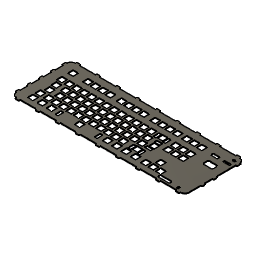
Plate v20 (Autodesk Fusion 360 design; units mm, degrees)
Autodesk Fusion 360 part; units mm, degrees
note: some values were not read from the file. Set by a fixed rule: which sketch regions a step uses.
(part 1 of 3)
sketch "Sketch1" plane through (0, 0, 0) normal (0, 0, 1) x (1, 0, 0)
  line L0 (3.025, -2.525) -> (16.025, -2.525)
  line L1 (3.025, -16.525) -> (16.025, -16.525)
  line L2 (2.525, -3.025) -> (2.525, -16.025)
  line L3 (16.525, -3.025) -> (16.525, -16.025)
  arc A0 (3.025, -2.525) -> (2.525, -3.025) centre (3.025, -3.025) ccw
  arc A1 (16.525, -3.025) -> (16.025, -2.525) centre (16.025, -3.025) ccw
  arc A2 (2.525, -16.025) -> (3.025, -16.525) centre (3.025, -16.025) ccw
  arc A3 (16.025, -16.525) -> (16.525, -16.025) centre (16.025, -16.025) ccw
  line L4 (41.125, -2.525) -> (54.125, -2.525)
  line L5 (41.125, -16.525) -> (54.125, -16.525)
  line L6 (40.625, -3.025) -> (40.625, -16.025)
  line L7 (54.625, -3.025) -> (54.625, -16.025)
  arc A4 (41.125, -2.525) -> (40.625, -3.025) centre (41.125, -3.025) ccw
  arc A5 (54.625, -3.025) -> (54.125, -2.525) centre (54.125, -3.025) ccw
  arc A6 (40.625, -16.025) -> (41.125, -16.525) centre (41.125, -16.025) ccw
  arc A7 (54.125, -16.525) -> (54.625, -16.025) centre (54.125, -16.025) ccw
  line L8 (60.175, -2.525) -> (73.175, -2.525)
  line L9 (60.175, -16.525) -> (73.175, -16.525)
  line L10 (59.675, -3.025) -> (59.675, -16.025)
  line L11 (73.675, -3.025) -> (73.675, -16.025)
  arc A8 (60.175, -2.525) -> (59.675, -3.025) centre (60.175, -3.025) ccw
  arc A9 (73.675, -3.025) -> (73.175, -2.525) centre (73.175, -3.025) ccw
  arc A10 (59.675, -16.025) -> (60.175, -16.525) centre (60.175, -16.025) ccw
  arc A11 (73.175, -16.525) -> (73.675, -16.025) centre (73.175, -16.025) ccw
  line L12 (79.225, -2.525) -> (92.225, -2.525)
  line L13 (79.225, -16.525) -> (92.225, -16.525)
  line L14 (78.725, -3.025) -> (78.725, -16.025)
  line L15 (92.725, -3.025) -> (92.725, -16.025)
  arc A12 (79.225, -2.525) -> (78.725, -3.025) centre (79.225, -3.025) ccw
  arc A13 (92.725, -3.025) -> (92.225, -2.525) centre (92.225, -3.025) ccw
  arc A14 (78.725, -16.025) -> (79.225, -16.525) centre (79.225, -16.025) ccw
  arc A15 (92.225, -16.525) -> (92.725, -16.025) centre (92.225, -16.025) ccw
  line L16 (98.275, -2.525) -> (111.275, -2.525)
  line L17 (98.275, -16.525) -> (111.275, -16.525)
  line L18 (97.775, -3.025) -> (97.775, -16.025)
  line L19 (111.775, -3.025) -> (111.775, -16.025)
  arc A16 (98.275, -2.525) -> (97.775, -3.025) centre (98.275, -3.025) ccw
  arc A17 (111.775, -3.025) -> (111.275, -2.525) centre (111.275, -3.025) ccw
  arc A18 (97.775, -16.025) -> (98.275, -16.525) centre (98.275, -16.025) ccw
  arc A19 (111.275, -16.525) -> (111.775, -16.025) centre (111.275, -16.025) ccw
  line L20 (126.85, -2.525) -> (139.85, -2.525)
  line L21 (126.85, -16.525) -> (139.85, -16.525)
  line L22 (126.35, -3.025) -> (126.35, -16.025)
  line L23 (140.35, -3.025) -> (140.35, -16.025)
  arc A20 (126.85, -2.525) -> (126.35, -3.025) centre (126.85, -3.025) ccw
  arc A21 (140.35, -3.025) -> (139.85, -2.525) centre (139.85, -3.025) ccw
  arc A22 (126.35, -16.025) -> (126.85, -16.525) centre (126.85, -16.025) ccw
  arc A23 (139.85, -16.525) -> (140.35, -16.025) centre (139.85, -16.025) ccw
  line L24 (145.9, -2.525) -> (158.9, -2.525)
  line L25 (145.9, -16.525) -> (158.9, -16.525)
  line L26 (145.4, -3.025) -> (145.4, -16.025)
  line L27 (159.4, -3.025) -> (159.4, -16.025)
  arc A24 (145.9, -2.525) -> (145.4, -3.025) centre (145.9, -3.025) ccw
  arc A25 (159.4, -3.025) -> (158.9, -2.525) centre (158.9, -3.025) ccw
  arc A26 (145.4, -16.025) -> (145.9, -16.525) centre (145.9, -16.025) ccw
  arc A27 (158.9, -16.525) -> (159.4, -16.025) centre (158.9, -16.025) ccw
  line L28 (164.95, -2.525) -> (177.95, -2.525)
  line L29 (164.95, -16.525) -> (177.95, -16.525)
  line L30 (164.45, -3.025) -> (164.45, -16.025)
  line L31 (178.45, -3.025) -> (178.45, -16.025)
  arc A28 (164.95, -2.525) -> (164.45, -3.025) centre (164.95, -3.025) ccw
  arc A29 (178.45, -3.025) -> (177.95, -2.525) centre (177.95, -3.025) ccw
  arc A30 (164.45, -16.025) -> (164.95, -16.525) centre (164.95, -16.025) ccw
  arc A31 (177.95, -16.525) -> (178.45, -16.025) centre (177.95, -16.025) ccw
  line L32 (184, -2.525) -> (197, -2.525)
  line L33 (184, -16.525) -> (197, -16.525)
  line L34 (183.5, -3.025) -> (183.5, -16.025)
  line L35 (197.5, -3.025) -> (197.5, -16.025)
  arc A32 (184, -2.525) -> (183.5, -3.025) centre (184, -3.025) ccw
  arc A33 (197.5, -3.025) -> (197, -2.525) centre (197, -3.025) ccw
  arc A34 (183.5, -16.025) -> (184, -16.525) centre (184, -16.025) ccw
  arc A35 (197, -16.525) -> (197.5, -16.025) centre (197, -16.025) ccw
  line L36 (212.575, -2.525) -> (225.575, -2.525)
  line L37 (212.575, -16.525) -> (225.575, -16.525)
  line L38 (212.075, -3.025) -> (212.075, -16.025)
  line L39 (226.075, -3.025) -> (226.075, -16.025)
  arc A36 (212.575, -2.525) -> (212.075, -3.025) centre (212.575, -3.025) ccw
  arc A37 (226.075, -3.025) -> (225.575, -2.525) centre (225.575, -3.025) ccw
  arc A38 (212.075, -16.025) -> (212.575, -16.525) centre (212.575, -16.025) ccw
  arc A39 (225.575, -16.525) -> (226.075, -16.025) centre (225.575, -16.025) ccw
  line L40 (231.625, -2.525) -> (244.625, -2.525)
  line L41 (231.625, -16.525) -> (244.625, -16.525)
  line L42 (231.125, -3.025) -> (231.125, -16.025)
  line L43 (245.125, -3.025) -> (245.125, -16.025)
  arc A40 (231.625, -2.525) -> (231.125, -3.025) centre (231.625, -3.025) ccw
  arc A41 (245.125, -3.025) -> (244.625, -2.525) centre (244.625, -3.025) ccw
  arc A42 (231.125, -16.025) -> (231.625, -16.525) centre (231.625, -16.025) ccw
  arc A43 (244.625, -16.525) -> (245.125, -16.025) centre (244.625, -16.025) ccw
  line L44 (250.675, -2.525) -> (263.675, -2.525)
  line L45 (250.675, -16.525) -> (263.675, -16.525)
  line L46 (250.175, -3.025) -> (250.175, -16.025)
  line L47 (264.175, -3.025) -> (264.175, -16.025)
  arc A44 (250.675, -2.525) -> (250.175, -3.025) centre (250.675, -3.025) ccw
  arc A45 (264.175, -3.025) -> (263.675, -2.525) centre (263.675, -3.025) ccw
  arc A46 (250.175, -16.025) -> (250.675, -16.525) centre (250.675, -16.025) ccw
  arc A47 (263.675, -16.525) -> (264.175, -16.025) centre (263.675, -16.025) ccw
  line L48 (269.725, -2.525) -> (282.725, -2.525)
  line L49 (269.725, -16.525) -> (282.725, -16.525)
  line L50 (269.225, -3.025) -> (269.225, -16.025)
  line L51 (283.225, -3.025) -> (283.225, -16.025)
  arc A48 (269.725, -2.525) -> (269.225, -3.025) centre (269.725, -3.025) ccw
  arc A49 (283.225, -3.025) -> (282.725, -2.525) centre (282.725, -3.025) ccw
  arc A50 (269.225, -16.025) -> (269.725, -16.525) centre (269.725, -16.025) ccw
  arc A51 (282.725, -16.525) -> (283.225, -16.025) centre (282.725, -16.025) ccw
  line L52 (293.5375, -2.525) -> (306.5375, -2.525)
  line L53 (293.5375, -16.525) -> (306.5375, -16.525)
  line L54 (293.0375, -3.025) -> (293.0375, -16.025)
  line L55 (307.0375, -3.025) -> (307.0375, -16.025)
  arc A52 (293.5375, -2.525) -> (293.0375, -3.025) centre (293.5375, -3.025) ccw
  arc A53 (307.0375, -3.025) -> (306.5375, -2.525) centre (306.5375, -3.025) ccw
  arc A54 (293.0375, -16.025) -> (293.5375, -16.525) centre (293.5375, -16.025) ccw
  arc A55 (306.5375, -16.525) -> (307.0375, -16.025) centre (306.5375, -16.025) ccw
  line L56 (312.5875, -2.525) -> (325.5875, -2.525)
  line L57 (312.5875, -16.525) -> (325.5875, -16.525)
  line L58 (312.0875, -3.025) -> (312.0875, -16.025)
  line L59 (326.0875, -3.025) -> (326.0875, -16.025)
  arc A56 (312.5875, -2.525) -> (312.0875, -3.025) centre (312.5875, -3.025) ccw
  arc A57 (326.0875, -3.025) -> (325.5875, -2.525) centre (325.5875, -3.025) ccw
  arc A58 (312.0875, -16.025) -> (312.5875, -16.525) centre (312.5875, -16.025) ccw
  arc A59 (325.5875, -16.525) -> (326.0875, -16.025) centre (325.5875, -16.025) ccw
  line L60 (331.6375, -2.525) -> (344.6375, -2.525)
  line L61 (331.6375, -16.525) -> (344.6375, -16.525)
  line L62 (331.1375, -3.025) -> (331.1375, -16.025)
  line L63 (345.1375, -3.025) -> (345.1375, -16.025)
  arc A60 (331.6375, -2.525) -> (331.1375, -3.025) centre (331.6375, -3.025) ccw
  arc A61 (345.1375, -3.025) -> (344.6375, -2.525) centre (344.6375, -3.025) ccw
  arc A62 (331.1375, -16.025) -> (331.6375, -16.525) centre (331.6375, -16.025) ccw
  arc A63 (344.6375, -16.525) -> (345.1375, -16.025) centre (344.6375, -16.025) ccw
  line L64 (3.025, -31.1) -> (16.025, -31.1)
  line L65 (3.025, -45.1) -> (16.025, -45.1)
  line L66 (2.525, -31.6) -> (2.525, -44.6)
  line L67 (16.525, -31.6) -> (16.525, -44.6)
  arc A64 (3.025, -31.1) -> (2.525, -31.6) centre (3.025, -31.6) ccw
  arc A65 (16.525, -31.6) -> (16.025, -31.1) centre (16.025, -31.6) ccw
  arc A66 (2.525, -44.6) -> (3.025, -45.1) centre (3.025, -44.6) ccw
  arc A67 (16.025, -45.1) -> (16.525, -44.6) centre (16.025, -44.6) ccw
  line L68 (22.075, -31.1) -> (35.075, -31.1)
  line L69 (22.075, -45.1) -> (35.075, -45.1)
  line L70 (21.575, -31.6) -> (21.575, -44.6)
  line L71 (35.575, -31.6) -> (35.575, -44.6)
  arc A68 (22.075, -31.1) -> (21.575, -31.6) centre (22.075, -31.6) ccw
  arc A69 (35.575, -31.6) -> (35.075, -31.1) centre (35.075, -31.6) ccw
  arc A70 (21.575, -44.6) -> (22.075, -45.1) centre (22.075, -44.6) ccw
  arc A71 (35.075, -45.1) -> (35.575, -44.6) centre (35.075, -44.6) ccw
  line L72 (41.125, -31.1) -> (54.125, -31.1)
  line L73 (41.125, -45.1) -> (54.125, -45.1)
  line L74 (40.625, -31.6) -> (40.625, -44.6)
  line L75 (54.625, -31.6) -> (54.625, -44.6)
  arc A72 (41.125, -31.1) -> (40.625, -31.6) centre (41.125, -31.6) ccw
  arc A73 (54.625, -31.6) -> (54.125, -31.1) centre (54.125, -31.6) ccw
  arc A74 (40.625, -44.6) -> (41.125, -45.1) centre (41.125, -44.6) ccw
  arc A75 (54.125, -45.1) -> (54.625, -44.6) centre (54.125, -44.6) ccw
  line L76 (60.175, -31.1) -> (73.175, -31.1)
  line L77 (60.175, -45.1) -> (73.175, -45.1)
  line L78 (59.675, -31.6) -> (59.675, -44.6)
  line L79 (73.675, -31.6) -> (73.675, -44.6)
  arc A76 (60.175, -31.1) -> (59.675, -31.6) centre (60.175, -31.6) ccw
  arc A77 (73.675, -31.6) -> (73.175, -31.1) centre (73.175, -31.6) ccw
  arc A78 (59.675, -44.6) -> (60.175, -45.1) centre (60.175, -44.6) ccw
  arc A79 (73.175, -45.1) -> (73.675, -44.6) centre (73.175, -44.6) ccw
  line L80 (79.225, -31.1) -> (92.225, -31.1)
  line L81 (79.225, -45.1) -> (92.225, -45.1)
  line L82 (78.725, -31.6) -> (78.725, -44.6)
  line L83 (92.725, -31.6) -> (92.725, -44.6)
  arc A80 (79.225, -31.1) -> (78.725, -31.6) centre (79.225, -31.6) ccw
  arc A81 (92.725, -31.6) -> (92.225, -31.1) centre (92.225, -31.6) ccw
  arc A82 (78.725, -44.6) -> (79.225, -45.1) centre (79.225, -44.6) ccw
  arc A83 (92.225, -45.1) -> (92.725, -44.6) centre (92.225, -44.6) ccw
  line L84 (98.275, -31.1) -> (111.275, -31.1)
  line L85 (98.275, -45.1) -> (111.275, -45.1)
  line L86 (97.775, -31.6) -> (97.775, -44.6)
  line L87 (111.775, -31.6) -> (111.775, -44.6)
  arc A84 (98.275, -31.1) -> (97.775, -31.6) centre (98.275, -31.6) ccw
  arc A85 (111.775, -31.6) -> (111.275, -31.1) centre (111.275, -31.6) ccw
  arc A86 (97.775, -44.6) -> (98.275, -45.1) centre (98.275, -44.6) ccw
  arc A87 (111.275, -45.1) -> (111.775, -44.6) centre (111.275, -44.6) ccw
  line L88 (117.325, -31.1) -> (130.325, -31.1)
  line L89 (117.325, -45.1) -> (130.325, -45.1)
  line L90 (116.825, -31.6) -> (116.825, -44.6)
  line L91 (130.825, -31.6) -> (130.825, -44.6)
  arc A88 (117.325, -31.1) -> (116.825, -31.6) centre (117.325, -31.6) ccw
  arc A89 (130.825, -31.6) -> (130.325, -31.1) centre (130.325, -31.6) ccw
  arc A90 (116.825, -44.6) -> (117.325, -45.1) centre (117.325, -44.6) ccw
  arc A91 (130.325, -45.1) -> (130.825, -44.6) centre (130.325, -44.6) ccw
  line L92 (136.375, -31.1) -> (149.375, -31.1)
  line L93 (136.375, -45.1) -> (149.375, -45.1)
  line L94 (135.875, -31.6) -> (135.875, -44.6)
  line L95 (149.875, -31.6) -> (149.875, -44.6)
  arc A92 (136.375, -31.1) -> (135.875, -31.6) centre (136.375, -31.6) ccw
  arc A93 (149.875, -31.6) -> (149.375, -31.1) centre (149.375, -31.6) ccw
  arc A94 (135.875, -44.6) -> (136.375, -45.1) centre (136.375, -44.6) ccw
  arc A95 (149.375, -45.1) -> (149.875, -44.6) centre (149.375, -44.6) ccw
  line L96 (155.425, -31.1) -> (168.425, -31.1)
  line L97 (155.425, -45.1) -> (168.425, -45.1)
  line L98 (154.925, -31.6) -> (154.925, -44.6)
  line L99 (168.925, -31.6) -> (168.925, -44.6)
  arc A96 (155.425, -31.1) -> (154.925, -31.6) centre (155.425, -31.6) ccw
  arc A97 (168.925, -31.6) -> (168.425, -31.1) centre (168.425, -31.6) ccw
  arc A98 (154.925, -44.6) -> (155.425, -45.1) centre (155.425, -44.6) ccw
  arc A99 (168.425, -45.1) -> (168.925, -44.6) centre (168.425, -44.6) ccw
  line L100 (174.475, -31.1) -> (187.475, -31.1)
  line L101 (174.475, -45.1) -> (187.475, -45.1)
  line L102 (173.975, -31.6) -> (173.975, -44.6)
  line L103 (187.975, -31.6) -> (187.975, -44.6)
  arc A100 (174.475, -31.1) -> (173.975, -31.6) centre (174.475, -31.6) ccw
  arc A101 (187.975, -31.6) -> (187.475, -31.1) centre (187.475, -31.6) ccw
  arc A102 (173.975, -44.6) -> (174.475, -45.1) centre (174.475, -44.6) ccw
  arc A103 (187.475, -45.1) -> (187.975, -44.6) centre (187.475, -44.6) ccw
  line L104 (193.525, -31.1) -> (206.525, -31.1)
  line L105 (193.525, -45.1) -> (206.525, -45.1)
  line L106 (193.025, -31.6) -> (193.025, -44.6)
  line L107 (207.025, -31.6) -> (207.025, -44.6)
  arc A104 (193.525, -31.1) -> (193.025, -31.6) centre (193.525, -31.6) ccw
  arc A105 (207.025, -31.6) -> (206.525, -31.1) centre (206.525, -31.6) ccw
  arc A106 (193.025, -44.6) -> (193.525, -45.1) centre (193.525, -44.6) ccw
  arc A107 (206.525, -45.1) -> (207.025, -44.6) centre (206.525, -44.6) ccw
  line L108 (212.575, -31.1) -> (225.575, -31.1)
  line L109 (212.575, -45.1) -> (225.575, -45.1)
  line L110 (212.075, -31.6) -> (212.075, -44.6)
  line L111 (226.075, -31.6) -> (226.075, -44.6)
  arc A108 (212.575, -31.1) -> (212.075, -31.6) centre (212.575, -31.6) ccw
  arc A109 (226.075, -31.6) -> (225.575, -31.1) centre (225.575, -31.6) ccw
  arc A110 (212.075, -44.6) -> (212.575, -45.1) centre (212.575, -44.6) ccw
  arc A111 (225.575, -45.1) -> (226.075, -44.6) centre (225.575, -44.6) ccw
  line L112 (231.625, -31.1) -> (244.625, -31.1)
  line L113 (231.625, -45.1) -> (244.625, -45.1)
  line L114 (231.125, -31.6) -> (231.125, -44.6)
  line L115 (245.125, -31.6) -> (245.125, -44.6)
  arc A112 (231.625, -31.1) -> (231.125, -31.6) centre (231.625, -31.6) ccw
  arc A113 (245.125, -31.6) -> (244.625, -31.1) centre (244.625, -31.6) ccw
  arc A114 (231.125, -44.6) -> (231.625, -45.1) centre (231.625, -44.6) ccw
  arc A115 (244.625, -45.1) -> (245.125, -44.6) centre (244.625, -44.6) ccw
  line L116 (260.2, -31.1) -> (273.2, -31.1)
  line L117 (260.2, -45.1) -> (273.2, -45.1)
  line L118 (259.7, -31.6) -> (259.7, -44.6)
  line L119 (273.7, -31.6) -> (273.7, -44.6)
  arc A116 (260.2, -31.1) -> (259.7, -31.6) centre (260.2, -31.6) ccw
  arc A117 (273.7, -31.6) -> (273.2, -31.1) centre (273.2, -31.6) ccw
  arc A118 (259.7, -44.6) -> (260.2, -45.1) centre (260.2, -44.6) ccw
  arc A119 (273.2, -45.1) -> (273.7, -44.6) centre (273.2, -44.6) ccw
  line L120 (251.762, -32.1) -> (257.762, -32.1)
  line L121 (251.762, -47.1) -> (257.762, -47.1)
  line L122 (251.262, -32.6) -> (251.262, -46.6)
  line L123 (258.262, -32.6) -> (258.262, -46.6)
  arc A120 (251.762, -32.1) -> (251.262, -32.6) centre (251.762, -32.6) ccw
  arc A121 (258.262, -32.6) -> (257.762, -32.1) centre (257.762, -32.6) ccw
  arc A122 (251.262, -46.6) -> (251.762, -47.1) centre (251.762, -46.6) ccw
  arc A123 (257.762, -47.1) -> (258.262, -46.6) centre (257.762, -46.6) ccw
  line L124 (275.638, -32.1) -> (281.638, -32.1)
  line L125 (275.638, -47.1) -> (281.638, -47.1)
  line L126 (275.138, -32.6) -> (275.138, -46.6)
  line L127 (282.138, -32.6) -> (282.138, -46.6)
  arc A124 (275.638, -32.1) -> (275.138, -32.6) centre (275.638, -32.6) ccw
  arc A125 (282.138, -32.6) -> (281.638, -32.1) centre (281.638, -32.6) ccw
  arc A126 (275.138, -46.6) -> (275.638, -47.1) centre (275.638, -46.6) ccw
  arc A127 (281.638, -47.1) -> (282.138, -46.6) centre (281.638, -46.6) ccw
  line L128 (293.5375, -31.1) -> (306.5375, -31.1)
  line L129 (293.5375, -45.1) -> (306.5375, -45.1)
  line L130 (293.0375, -31.6) -> (293.0375, -44.6)
  line L131 (307.0375, -31.6) -> (307.0375, -44.6)
  arc A128 (293.5375, -31.1) -> (293.0375, -31.6) centre (293.5375, -31.6) ccw
  arc A129 (307.0375, -31.6) -> (306.5375, -31.1) centre (306.5375, -31.6) ccw
  arc A130 (293.0375, -44.6) -> (293.5375, -45.1) centre (293.5375, -44.6) ccw
  arc A131 (306.5375, -45.1) -> (307.0375, -44.6) centre (306.5375, -44.6) ccw
  line L132 (312.5875, -31.1) -> (325.5875, -31.1)
  line L133 (312.5875, -45.1) -> (325.5875, -45.1)
  line L134 (312.0875, -31.6) -> (312.0875, -44.6)
  line L135 (326.0875, -31.6) -> (326.0875, -44.6)
  arc A132 (312.5875, -31.1) -> (312.0875, -31.6) centre (312.5875, -31.6) ccw
  arc A133 (326.0875, -31.6) -> (325.5875, -31.1) centre (325.5875, -31.6) ccw
  arc A134 (312.0875, -44.6) -> (312.5875, -45.1) centre (312.5875, -44.6) ccw
  arc A135 (325.5875, -45.1) -> (326.0875, -44.6) centre (325.5875, -44.6) ccw
  line L136 (331.6375, -31.1) -> (344.6375, -31.1)
  line L137 (331.6375, -45.1) -> (344.6375, -45.1)
  line L138 (331.1375, -31.6) -> (331.1375, -44.6)
  line L139 (345.1375, -31.6) -> (345.1375, -44.6)
  arc A136 (331.6375, -31.1) -> (331.1375, -31.6) centre (331.6375, -31.6) ccw
  arc A137 (345.1375, -31.6) -> (344.6375, -31.1) centre (344.6375, -31.6) ccw
  arc A138 (331.1375, -44.6) -> (331.6375, -45.1) centre (331.6375, -44.6) ccw
  arc A139 (344.6375, -45.1) -> (345.1375, -44.6) centre (344.6375, -44.6) ccw
  line L140 (7.7875, -50.15) -> (20.7875, -50.15)
  line L141 (7.7875, -64.15) -> (20.7875, -64.15)
  line L142 (7.2875, -50.65) -> (7.2875, -63.65)
  line L143 (21.2875, -50.65) -> (21.2875, -63.65)
  arc A140 (7.7875, -50.15) -> (7.2875, -50.65) centre (7.7875, -50.65) ccw
  arc A141 (21.2875, -50.65) -> (20.7875, -50.15) centre (20.7875, -50.65) ccw
  arc A142 (7.2875, -63.65) -> (7.7875, -64.15) centre (7.7875, -63.65) ccw
  arc A143 (20.7875, -64.15) -> (21.2875, -63.65) centre (20.7875, -63.65) ccw
  line L144 (31.6, -50.15) -> (44.6, -50.15)
  line L145 (31.6, -64.15) -> (44.6, -64.15)
  line L146 (31.1, -50.65) -> (31.1, -63.65)
  line L147 (45.1, -50.65) -> (45.1, -63.65)
  arc A144 (31.6, -50.15) -> (31.1, -50.65) centre (31.6, -50.65) ccw
  arc A145 (45.1, -50.65) -> (44.6, -50.15) centre (44.6, -50.65) ccw
  arc A146 (31.1, -63.65) -> (31.6, -64.15) centre (31.6, -63.65) ccw
  arc A147 (44.6, -64.15) -> (45.1, -63.65) centre (44.6, -63.65) ccw
  line L148 (50.65, -50.15) -> (63.65, -50.15)
  line L149 (50.65, -64.15) -> (63.65, -64.15)
  line L150 (50.15, -50.65) -> (50.15, -63.65)
  line L151 (64.15, -50.65) -> (64.15, -63.65)
  arc A148 (50.65, -50.15) -> (50.15, -50.65) centre (50.65, -50.65) ccw
  arc A149 (64.15, -50.65) -> (63.65, -50.15) centre (63.65, -50.65) ccw
  arc A150 (50.15, -63.65) -> (50.65, -64.15) centre (50.65, -63.65) ccw
  arc A151 (63.65, -64.15) -> (64.15, -63.65) centre (63.65, -63.65) ccw
  line L152 (69.7, -50.15) -> (82.7, -50.15)
  line L153 (69.7, -64.15) -> (82.7, -64.15)
  line L154 (69.2, -50.65) -> (69.2, -63.65)
  line L155 (83.2, -50.65) -> (83.2, -63.65)
  arc A152 (69.7, -50.15) -> (69.2, -50.65) centre (69.7, -50.65) ccw
  arc A153 (83.2, -50.65) -> (82.7, -50.15) centre (82.7, -50.65) ccw
  arc A154 (69.2, -63.65) -> (69.7, -64.15) centre (69.7, -63.65) ccw
  arc A155 (82.7, -64.15) -> (83.2, -63.65) centre (82.7, -63.65) ccw
  line L156 (88.75, -50.15) -> (101.75, -50.15)
  line L157 (88.75, -64.15) -> (101.75, -64.15)
  line L158 (88.25, -50.65) -> (88.25, -63.65)
  line L159 (102.25, -50.65) -> (102.25, -63.65)
  arc A156 (88.75, -50.15) -> (88.25, -50.65) centre (88.75, -50.65) ccw
  arc A157 (102.25, -50.65) -> (101.75, -50.15) centre (101.75, -50.65) ccw
  arc A158 (88.25, -63.65) -> (88.75, -64.15) centre (88.75, -63.65) ccw
  arc A159 (101.75, -64.15) -> (102.25, -63.65) centre (101.75, -63.65) ccw
  line L160 (107.8, -50.15) -> (120.8, -50.15)
  line L161 (107.8, -64.15) -> (120.8, -64.15)
  line L162 (107.3, -50.65) -> (107.3, -63.65)
  line L163 (121.3, -50.65) -> (121.3, -63.65)
  arc A160 (107.8, -50.15) -> (107.3, -50.65) centre (107.8, -50.65) ccw
  arc A161 (121.3, -50.65) -> (120.8, -50.15) centre (120.8, -50.65) ccw
  arc A162 (107.3, -63.65) -> (107.8, -64.15) centre (107.8, -63.65) ccw
  arc A163 (120.8, -64.15) -> (121.3, -63.65) centre (120.8, -63.65) ccw
  line L164 (126.85, -50.15) -> (139.85, -50.15)
  line L165 (126.85, -64.15) -> (139.85, -64.15)
  line L166 (126.35, -50.65) -> (126.35, -63.65)
  line L167 (140.35, -50.65) -> (140.35, -63.65)
  arc A164 (126.85, -50.15) -> (126.35, -50.65) centre (126.85, -50.65) ccw
  arc A165 (140.35, -50.65) -> (139.85, -50.15) centre (139.85, -50.65) ccw
  arc A166 (126.35, -63.65) -> (126.85, -64.15) centre (126.85, -63.65) ccw
  arc A167 (139.85, -64.15) -> (140.35, -63.65) centre (139.85, -63.65) ccw
  line L168 (145.9, -50.15) -> (158.9, -50.15)
  line L169 (145.9, -64.15) -> (158.9, -64.15)
  line L170 (145.4, -50.65) -> (145.4, -63.65)
  line L171 (159.4, -50.65) -> (159.4, -63.65)
  arc A168 (145.9, -50.15) -> (145.4, -50.65) centre (145.9, -50.65) ccw
  arc A169 (159.4, -50.65) -> (158.9, -50.15) centre (158.9, -50.65) ccw
  arc A170 (145.4, -63.65) -> (145.9, -64.15) centre (145.9, -63.65) ccw
  arc A171 (158.9, -64.15) -> (159.4, -63.65) centre (158.9, -63.65) ccw
  line L172 (164.95, -50.15) -> (177.95, -50.15)
  line L173 (164.95, -64.15) -> (177.95, -64.15)
  line L174 (164.45, -50.65) -> (164.45, -63.65)
  line L175 (178.45, -50.65) -> (178.45, -63.65)
  arc A172 (164.95, -50.15) -> (164.45, -50.65) centre (164.95, -50.65) ccw
  arc A173 (178.45, -50.65) -> (177.95, -50.15) centre (177.95, -50.65) ccw
  arc A174 (164.45, -63.65) -> (164.95, -64.15) centre (164.95, -63.65) ccw
  arc A175 (177.95, -64.15) -> (178.45, -63.65) centre (177.95, -63.65) ccw
  line L176 (184, -50.15) -> (197, -50.15)
  line L177 (184, -64.15) -> (197, -64.15)
  line L178 (183.5, -50.65) -> (183.5, -63.65)
  line L179 (197.5, -50.65) -> (197.5, -63.65)
  arc A176 (184, -50.15) -> (183.5, -50.65) centre (184, -50.65) ccw
  arc A177 (197.5, -50.65) -> (197, -50.15) centre (197, -50.65) ccw
  arc A178 (183.5, -63.65) -> (184, -64.15) centre (184, -63.65) ccw
  arc A179 (197, -64.15) -> (197.5, -63.65) centre (197, -63.65) ccw
  line L180 (203.05, -50.15) -> (216.05, -50.15)
  line L181 (203.05, -64.15) -> (216.05, -64.15)
  line L182 (202.55, -50.65) -> (202.55, -63.65)
  line L183 (216.55, -50.65) -> (216.55, -63.65)
  arc A180 (203.05, -50.15) -> (202.55, -50.65) centre (203.05, -50.65) ccw
  arc A181 (216.55, -50.65) -> (216.05, -50.15) centre (216.05, -50.65) ccw
  arc A182 (202.55, -63.65) -> (203.05, -64.15) centre (203.05, -63.65) ccw
  arc A183 (216.05, -64.15) -> (216.55, -63.65) centre (216.05, -63.65) ccw
  line L184 (222.1, -50.15) -> (235.1, -50.15)
  line L185 (222.1, -64.15) -> (235.1, -64.15)
  line L186 (221.6, -50.65) -> (221.6, -63.65)
  line L187 (235.6, -50.65) -> (235.6, -63.65)
  arc A184 (222.1, -50.15) -> (221.6, -50.65) centre (222.1, -50.65) ccw
  arc A185 (235.6, -50.65) -> (235.1, -50.15) centre (235.1, -50.65) ccw
  arc A186 (221.6, -63.65) -> (222.1, -64.15) centre (222.1, -63.65) ccw
  arc A187 (235.1, -64.15) -> (235.6, -63.65) centre (235.1, -63.65) ccw
  line L188 (241.15, -50.15) -> (254.15, -50.15)
  line L189 (241.15, -64.15) -> (254.15, -64.15)
  line L190 (240.65, -50.65) -> (240.65, -63.65)
  line L191 (254.65, -50.65) -> (254.65, -63.65)
  arc A188 (241.15, -50.15) -> (240.65, -50.65) centre (241.15, -50.65) ccw
  arc A189 (254.65, -50.65) -> (254.15, -50.15) centre (254.15, -50.65) ccw
  arc A190 (240.65, -63.65) -> (241.15, -64.15) centre (241.15, -63.65) ccw
  arc A191 (254.15, -64.15) -> (254.65, -63.65) centre (254.15, -63.65) ccw
  line L192 (280.8438, -60.175) -> (280.8438, -73.175)
  line L193 (266.8438, -60.175) -> (266.8438, -73.175)
  line L194 (280.3438, -59.675) -> (267.3438, -59.675)
  line L195 (280.3438, -73.675) -> (267.3438, -73.675)
  arc A192 (280.8438, -60.175) -> (280.3438, -59.675) centre (280.3438, -60.175) ccw
  arc A193 (280.3438, -73.675) -> (280.8438, -73.175) centre (280.3438, -73.175) ccw
  arc A194 (267.3438, -59.675) -> (266.8438, -60.175) centre (267.3438, -60.175) ccw
  arc A195 (266.8438, -73.175) -> (267.3438, -73.675) centre (267.3438, -73.175) ccw
  line L196 (279.8438, -51.737) -> (279.8438, -57.737)
  line L197 (264.8438, -51.737) -> (264.8438, -57.737)
  line L198 (279.3438, -51.237) -> (265.3438, -51.237)
  line L199 (279.3438, -58.237) -> (265.3438, -58.237)
  arc A196 (279.8438, -51.737) -> (279.3438, -51.237) centre (279.3438, -51.737) ccw
  arc A197 (279.3438, -58.237) -> (279.8438, -57.737) centre (279.3438, -57.737) ccw
  arc A198 (265.3438, -51.237) -> (264.8438, -51.737) centre (265.3438, -51.737) ccw
  arc A199 (264.8438, -57.737) -> (265.3438, -58.237) centre (265.3438, -57.737) ccw
  line L200 (279.8438, -75.613) -> (279.8438, -81.613)
  line L201 (264.8438, -75.613) -> (264.8438, -81.613)
  line L202 (279.3438, -75.113) -> (265.3438, -75.113)
  line L203 (279.3438, -82.113) -> (265.3438, -82.113)
  arc A200 (279.8438, -75.613) -> (279.3438, -75.113) centre (279.3438, -75.613) ccw
  arc A201 (279.3438, -82.113) -> (279.8438, -81.613) centre (279.3438, -81.613) ccw
  arc A202 (265.3438, -75.113) -> (264.8438, -75.613) centre (265.3438, -75.613) ccw
  arc A203 (264.8438, -81.613) -> (265.3438, -82.113) centre (265.3438, -81.613) ccw
  line L204 (293.5375, -50.15) -> (306.5375, -50.15)
  line L205 (293.5375, -64.15) -> (306.5375, -64.15)
  line L206 (293.0375, -50.65) -> (293.0375, -63.65)
  line L207 (307.0375, -50.65) -> (307.0375, -63.65)
  arc A204 (293.5375, -50.15) -> (293.0375, -50.65) centre (293.5375, -50.65) ccw
  arc A205 (307.0375, -50.65) -> (306.5375, -50.15) centre (306.5375, -50.65) ccw
  arc A206 (293.0375, -63.65) -> (293.5375, -64.15) centre (293.5375, -63.65) ccw
  arc A207 (306.5375, -64.15) -> (307.0375, -63.65) centre (306.5375, -63.65) ccw
  line L208 (312.5875, -50.15) -> (325.5875, -50.15)
  line L209 (312.5875, -64.15) -> (325.5875, -64.15)
  line L210 (312.0875, -50.65) -> (312.0875, -63.65)
  line L211 (326.0875, -50.65) -> (326.0875, -63.65)
  arc A208 (312.5875, -50.15) -> (312.0875, -50.65) centre (312.5875, -50.65) ccw
  arc A209 (326.0875, -50.65) -> (325.5875, -50.15) centre (325.5875, -50.65) ccw
  arc A210 (312.0875, -63.65) -> (312.5875, -64.15) centre (312.5875, -63.65) ccw
  arc A211 (325.5875, -64.15) -> (326.0875, -63.65) centre (325.5875, -63.65) ccw
  line L212 (331.6375, -50.15) -> (344.6375, -50.15)
  line L213 (331.6375, -64.15) -> (344.6375, -64.15)
  line L214 (331.1375, -50.65) -> (331.1375, -63.65)
  line L215 (345.1375, -50.65) -> (345.1375, -63.65)
  arc A212 (331.6375, -50.15) -> (331.1375, -50.65) centre (331.6375, -50.65) ccw
  arc A213 (345.1375, -50.65) -> (344.6375, -50.15) centre (344.6375, -50.65) ccw
  arc A214 (331.1375, -63.65) -> (331.6375, -64.15) centre (331.6375, -63.65) ccw
  arc A215 (344.6375, -64.15) -> (345.1375, -63.65) centre (344.6375, -63.65) ccw
  line L216 (10.1687, -69.2) -> (23.1687, -69.2)
  line L217 (10.1687, -83.2) -> (23.1687, -83.2)
  line L218 (9.6687, -69.7) -> (9.6687, -82.7)
  line L219 (23.6687, -69.7) -> (23.6687, -82.7)
  arc A216 (10.1687, -69.2) -> (9.6688, -69.7) centre (10.1687, -69.7) ccw
  arc A217 (23.6687, -69.7) -> (23.1687, -69.2) centre (23.1687, -69.7) ccw
  arc A218 (9.6687, -82.7) -> (10.1687, -83.2) centre (10.1687, -82.7) ccw
  arc A219 (23.1687, -83.2) -> (23.6687, -82.7) centre (23.1687, -82.7) ccw
  line L220 (36.3625, -69.2) -> (49.3625, -69.2)
  line L221 (36.3625, -83.2) -> (49.3625, -83.2)
  line L222 (35.8625, -69.7) -> (35.8625, -82.7)
  line L223 (49.8625, -69.7) -> (49.8625, -82.7)
  arc A220 (36.3625, -69.2) -> (35.8625, -69.7) centre (36.3625, -69.7) ccw
  arc A221 (49.8625, -69.7) -> (49.3625, -69.2) centre (49.3625, -69.7) ccw
  arc A222 (35.8625, -82.7) -> (36.3625, -83.2) centre (36.3625, -82.7) ccw
  arc A223 (49.3625, -83.2) -> (49.8625, -82.7) centre (49.3625, -82.7) ccw
  line L224 (55.4125, -69.2) -> (68.4125, -69.2)
  line L225 (55.4125, -83.2) -> (68.4125, -83.2)
  line L226 (54.9125, -69.7) -> (54.9125, -82.7)
  line L227 (68.9125, -69.7) -> (68.9125, -82.7)
  arc A224 (55.4125, -69.2) -> (54.9125, -69.7) centre (55.4125, -69.7) ccw
  arc A225 (68.9125, -69.7) -> (68.4125, -69.2) centre (68.4125, -69.7) ccw
  arc A226 (54.9125, -82.7) -> (55.4125, -83.2) centre (55.4125, -82.7) ccw
  arc A227 (68.4125, -83.2) -> (68.9125, -82.7) centre (68.4125, -82.7) ccw
  line L228 (74.4625, -69.2) -> (87.4625, -69.2)
  line L229 (74.4625, -83.2) -> (87.4625, -83.2)
  line L230 (73.9625, -69.7) -> (73.9625, -82.7)
  line L231 (87.9625, -69.7) -> (87.9625, -82.7)
  arc A228 (74.4625, -69.2) -> (73.9625, -69.7) centre (74.4625, -69.7) ccw
  arc A229 (87.9625, -69.7) -> (87.4625, -69.2) centre (87.4625, -69.7) ccw
  arc A230 (73.9625, -82.7) -> (74.4625, -83.2) centre (74.4625, -82.7) ccw
  arc A231 (87.4625, -83.2) -> (87.9625, -82.7) centre (87.4625, -82.7) ccw
  line L232 (93.5125, -69.2) -> (106.5125, -69.2)
  line L233 (93.5125, -83.2) -> (106.5125, -83.2)
  line L234 (93.0125, -69.7) -> (93.0125, -82.7)
  line L235 (107.0125, -69.7) -> (107.0125, -82.7)
  arc A232 (93.5125, -69.2) -> (93.0125, -69.7) centre (93.5125, -69.7) ccw
  arc A233 (107.0125, -69.7) -> (106.5125, -69.2) centre (106.5125, -69.7) ccw
  arc A234 (93.0125, -82.7) -> (93.5125, -83.2) centre (93.5125, -82.7) ccw
  arc A235 (106.5125, -83.2) -> (107.0125, -82.7) centre (106.5125, -82.7) ccw
  line L236 (112.5625, -69.2) -> (125.5625, -69.2)
  line L237 (112.5625, -83.2) -> (125.5625, -83.2)
  line L238 (112.0625, -69.7) -> (112.0625, -82.7)
  line L239 (126.0625, -69.7) -> (126.0625, -82.7)
  arc A236 (112.5625, -69.2) -> (112.0625, -69.7) centre (112.5625, -69.7) ccw
  arc A237 (126.0625, -69.7) -> (125.5625, -69.2) centre (125.5625, -69.7) ccw
  arc A238 (112.0625, -82.7) -> (112.5625, -83.2) centre (112.5625, -82.7) ccw
  arc A239 (125.5625, -83.2) -> (126.0625, -82.7) centre (125.5625, -82.7) ccw
  line L240 (131.6125, -69.2) -> (144.6125, -69.2)
  line L241 (131.6125, -83.2) -> (144.6125, -83.2)
  line L242 (131.1125, -69.7) -> (131.1125, -82.7)
  line L243 (145.1125, -69.7) -> (145.1125, -82.7)
  arc A240 (131.6125, -69.2) -> (131.1125, -69.7) centre (131.6125, -69.7) ccw
  arc A241 (145.1125, -69.7) -> (144.6125, -69.2) centre (144.6125, -69.7) ccw
  arc A242 (131.1125, -82.7) -> (131.6125, -83.2) centre (131.6125, -82.7) ccw
  arc A243 (144.6125, -83.2) -> (145.1125, -82.7) centre (144.6125, -82.7) ccw
  line L244 (150.6625, -69.2) -> (163.6625, -69.2)
  line L245 (150.6625, -83.2) -> (163.6625, -83.2)
  line L246 (150.1625, -69.7) -> (150.1625, -82.7)
  line L247 (164.1625, -69.7) -> (164.1625, -82.7)
  arc A244 (150.6625, -69.2) -> (150.1625, -69.7) centre (150.6625, -69.7) ccw
  arc A245 (164.1625, -69.7) -> (163.6625, -69.2) centre (163.6625, -69.7) ccw
  arc A246 (150.1625, -82.7) -> (150.6625, -83.2) centre (150.6625, -82.7) ccw
  arc A247 (163.6625, -83.2) -> (164.1625, -82.7) centre (163.6625, -82.7) ccw
  line L248 (169.7125, -69.2) -> (182.7125, -69.2)
  line L249 (169.7125, -83.2) -> (182.7125, -83.2)
  line L250 (169.2125, -69.7) -> (169.2125, -82.7)
  line L251 (183.2125, -69.7) -> (183.2125, -82.7)
  arc A248 (169.7125, -69.2) -> (169.2125, -69.7) centre (169.7125, -69.7) ccw
  arc A249 (183.2125, -69.7) -> (182.7125, -69.2) centre (182.7125, -69.7) ccw
  arc A250 (169.2125, -82.7) -> (169.7125, -83.2) centre (169.7125, -82.7) ccw
  arc A251 (182.7125, -83.2) -> (183.2125, -82.7) centre (182.7125, -82.7) ccw
  line L252 (188.7625, -69.2) -> (201.7625, -69.2)
  line L253 (188.7625, -83.2) -> (201.7625, -83.2)
  line L254 (188.2625, -69.7) -> (188.2625, -82.7)
  line L255 (202.2625, -69.7) -> (202.2625, -82.7)
  arc A252 (188.7625, -69.2) -> (188.2625, -69.7) centre (188.7625, -69.7) ccw
  arc A253 (202.2625, -69.7) -> (201.7625, -69.2) centre (201.7625, -69.7) ccw
  arc A254 (188.2625, -82.7) -> (188.7625, -83.2) centre (188.7625, -82.7) ccw
  arc A255 (201.7625, -83.2) -> (202.2625, -82.7) centre (201.7625, -82.7) ccw
  line L256 (207.8125, -69.2) -> (220.8125, -69.2)
  line L257 (207.8125, -83.2) -> (220.8125, -83.2)
  line L258 (207.3125, -69.7) -> (207.3125, -82.7)
  line L259 (221.3125, -69.7) -> (221.3125, -82.7)
  arc A256 (207.8125, -69.2) -> (207.3125, -69.7) centre (207.8125, -69.7) ccw
  arc A257 (221.3125, -69.7) -> (220.8125, -69.2) centre (220.8125, -69.7) ccw
  arc A258 (207.3125, -82.7) -> (207.8125, -83.2) centre (207.8125, -82.7) ccw
  arc A259 (220.8125, -83.2) -> (221.3125, -82.7) centre (220.8125, -82.7) ccw
  line L260 (226.8625, -69.2) -> (239.8625, -69.2)
  line L261 (226.8625, -83.2) -> (239.8625, -83.2)
  line L262 (226.3625, -69.7) -> (226.3625, -82.7)
  line L263 (240.3625, -69.7) -> (240.3625, -82.7)
  arc A260 (226.8625, -69.2) -> (226.3625, -69.7) centre (226.8625, -69.7) ccw
  arc A261 (240.3625, -69.7) -> (239.8625, -69.2) centre (239.8625, -69.7) ccw
  arc A262 (226.3625, -82.7) -> (226.8625, -83.2) centre (226.8625, -82.7) ccw
  arc A263 (239.8625, -83.2) -> (240.3625, -82.7) centre (239.8625, -82.7) ccw
  line L264 (245.9125, -69.2) -> (258.9125, -69.2)
  line L265 (245.9125, -83.2) -> (258.9125, -83.2)
  line L266 (245.4125, -69.7) -> (245.4125, -82.7)
  line L267 (259.4125, -69.7) -> (259.4125, -82.7)
  arc A264 (245.9125, -69.2) -> (245.4125, -69.7) centre (245.9125, -69.7) ccw
  arc A265 (259.4125, -69.7) -> (258.9125, -69.2) centre (258.9125, -69.7) ccw
  arc A266 (245.4125, -82.7) -> (245.9125, -83.2) centre (245.9125, -82.7) ccw
  arc A267 (258.9125, -83.2) -> (259.4125, -82.7) centre (258.9125, -82.7) ccw
  line L268 (5.4062, -88.25) -> (18.4063, -88.25)
  line L269 (5.4062, -102.25) -> (18.4063, -102.25)
  line L270 (4.9062, -88.75) -> (4.9062, -101.75)
  line L271 (18.9062, -88.75) -> (18.9062, -101.75)
  arc A268 (5.4062, -88.25) -> (4.9063, -88.75) centre (5.4062, -88.75) ccw
  arc A269 (18.9062, -88.75) -> (18.4062, -88.25) centre (18.4062, -88.75) ccw
  arc A270 (4.9062, -101.75) -> (5.4062, -102.25) centre (5.4062, -101.75) ccw
  arc A271 (18.4062, -102.25) -> (18.9063, -101.75) centre (18.4062, -101.75) ccw
  line L272 (26.8375, -88.25) -> (39.8375, -88.25)
  line L273 (26.8375, -102.25) -> (39.8375, -102.25)
  line L274 (26.3375, -88.75) -> (26.3375, -101.75)
  line L275 (40.3375, -88.75) -> (40.3375, -101.75)
  arc A272 (26.8375, -88.25) -> (26.3375, -88.75) centre (26.8375, -88.75) ccw
  arc A273 (40.3375, -88.75) -> (39.8375, -88.25) centre (39.8375, -88.75) ccw
  arc A274 (26.3375, -101.75) -> (26.8375, -102.25) centre (26.8375, -101.75) ccw
  arc A275 (39.8375, -102.25) -> (40.3375, -101.75) centre (39.8375, -101.75) ccw
  line L276 (45.8875, -88.25) -> (58.8875, -88.25)
  line L277 (45.8875, -102.25) -> (58.8875, -102.25)
  line L278 (45.3875, -88.75) -> (45.3875, -101.75)
  line L279 (59.3875, -88.75) -> (59.3875, -101.75)
  arc A276 (45.8875, -88.25) -> (45.3875, -88.75) centre (45.8875, -88.75) ccw
  arc A277 (59.3875, -88.75) -> (58.8875, -88.25) centre (58.8875, -88.75) ccw
  arc A278 (45.3875, -101.75) -> (45.8875, -102.25) centre (45.8875, -101.75) ccw
  arc A279 (58.8875, -102.25) -> (59.3875, -101.75) centre (58.8875, -101.75) ccw
  line L280 (64.9375, -88.25) -> (77.9375, -88.25)
  line L281 (64.9375, -102.25) -> (77.9375, -102.25)
  line L282 (64.4375, -88.75) -> (64.4375, -101.75)
  line L283 (78.4375, -88.75) -> (78.4375, -101.75)
  arc A280 (64.9375, -88.25) -> (64.4375, -88.75) centre (64.9375, -88.75) ccw
  arc A281 (78.4375, -88.75) -> (77.9375, -88.25) centre (77.9375, -88.75) ccw
  arc A282 (64.4375, -101.75) -> (64.9375, -102.25) centre (64.9375, -101.75) ccw
  arc A283 (77.9375, -102.25) -> (78.4375, -101.75) centre (77.9375, -101.75) ccw
  line L284 (83.9875, -88.25) -> (96.9875, -88.25)
  line L285 (83.9875, -102.25) -> (96.9875, -102.25)
  line L286 (83.4875, -88.75) -> (83.4875, -101.75)
  line L287 (97.4875, -88.75) -> (97.4875, -101.75)
  arc A284 (83.9875, -88.25) -> (83.4875, -88.75) centre (83.9875, -88.75) ccw
  arc A285 (97.4875, -88.75) -> (96.9875, -88.25) centre (96.9875, -88.75) ccw
  arc A286 (83.4875, -101.75) -> (83.9875, -102.25) centre (83.9875, -101.75) ccw
  arc A287 (96.9875, -102.25) -> (97.4875, -101.75) centre (96.9875, -101.75) ccw
  line L288 (103.0375, -88.25) -> (116.0375, -88.25)
  line L289 (103.0375, -102.25) -> (116.0375, -102.25)
  line L290 (102.5375, -88.75) -> (102.5375, -101.75)
  line L291 (116.5375, -88.75) -> (116.5375, -101.75)
  arc A288 (103.0375, -88.25) -> (102.5375, -88.75) centre (103.0375, -88.75) ccw
  arc A289 (116.5375, -88.75) -> (116.0375, -88.25) centre (116.0375, -88.75) ccw
  arc A290 (102.5375, -101.75) -> (103.0375, -102.25) centre (103.0375, -101.75) ccw
  arc A291 (116.0375, -102.25) -> (116.5375, -101.75) centre (116.0375, -101.75) ccw
  line L292 (122.0875, -88.25) -> (135.0875, -88.25)
  line L293 (122.0875, -102.25) -> (135.0875, -102.25)
  line L294 (121.5875, -88.75) -> (121.5875, -101.75)
  line L295 (135.5875, -88.75) -> (135.5875, -101.75)
  arc A292 (122.0875, -88.25) -> (121.5875, -88.75) centre (122.0875, -88.75) ccw
  arc A293 (135.5875, -88.75) -> (135.0875, -88.25) centre (135.0875, -88.75) ccw
  arc A294 (121.5875, -101.75) -> (122.0875, -102.25) centre (122.0875, -101.75) ccw
  arc A295 (135.0875, -102.25) -> (135.5875, -101.75) centre (135.0875, -101.75) ccw
  line L296 (141.1375, -88.25) -> (154.1375, -88.25)
  line L297 (141.1375, -102.25) -> (154.1375, -102.25)
  line L298 (140.6375, -88.75) -> (140.6375, -101.75)
  line L299 (154.6375, -88.75) -> (154.6375, -101.75)
  arc A296 (141.1375, -88.25) -> (140.6375, -88.75) centre (141.1375, -88.75) ccw
  arc A297 (154.6375, -88.75) -> (154.1375, -88.25) centre (154.1375, -88.75) ccw
  arc A298 (140.6375, -101.75) -> (141.1375, -102.25) centre (141.1375, -101.75) ccw
  arc A299 (154.1375, -102.25) -> (154.6375, -101.75) centre (154.1375, -101.75) ccw
  line L300 (160.1875, -88.25) -> (173.1875, -88.25)
  line L301 (160.1875, -102.25) -> (173.1875, -102.25)
  line L302 (159.6875, -88.75) -> (159.6875, -101.75)
  line L303 (173.6875, -88.75) -> (173.6875, -101.75)
  arc A300 (160.1875, -88.25) -> (159.6875, -88.75) centre (160.1875, -88.75) ccw
  arc A301 (173.6875, -88.75) -> (173.1875, -88.25) centre (173.1875, -88.75) ccw
  arc A302 (159.6875, -101.75) -> (160.1875, -102.25) centre (160.1875, -101.75) ccw
  arc A303 (173.1875, -102.25) -> (173.6875, -101.75) centre (173.1875, -101.75) ccw
  line L304 (179.2375, -88.25) -> (192.2375, -88.25)
  line L305 (179.2375, -102.25) -> (192.2375, -102.25)
  line L306 (178.7375, -88.75) -> (178.7375, -101.75)
  line L307 (192.7375, -88.75) -> (192.7375, -101.75)
  arc A304 (179.2375, -88.25) -> (178.7375, -88.75) centre (179.2375, -88.75) ccw
  arc A305 (192.7375, -88.75) -> (192.2375, -88.25) centre (192.2375, -88.75) ccw
  arc A306 (178.7375, -101.75) -> (179.2375, -102.25) centre (179.2375, -101.75) ccw
  arc A307 (192.2375, -102.25) -> (192.7375, -101.75) centre (192.2375, -101.75) ccw
  line L308 (198.2875, -88.25) -> (211.2875, -88.25)
  line L309 (198.2875, -102.25) -> (211.2875, -102.25)
  line L310 (197.7875, -88.75) -> (197.7875, -101.75)
  line L311 (211.7875, -88.75) -> (211.7875, -101.75)
  arc A308 (198.2875, -88.25) -> (197.7875, -88.75) centre (198.2875, -88.75) ccw
  arc A309 (211.7875, -88.75) -> (211.2875, -88.25) centre (211.2875, -88.75) ccw
  arc A310 (197.7875, -101.75) -> (198.2875, -102.25) centre (198.2875, -101.75) ccw
  arc A311 (211.2875, -102.25) -> (211.7875, -101.75) centre (211.2875, -101.75) ccw
  line L312 (217.3375, -88.25) -> (230.3375, -88.25)
  line L313 (217.3375, -102.25) -> (230.3375, -102.25)
  line L314 (216.8375, -88.75) -> (216.8375, -101.75)
  line L315 (230.8375, -88.75) -> (230.8375, -101.75)
  arc A312 (217.3375, -88.25) -> (216.8375, -88.75) centre (217.3375, -88.75) ccw
  arc A313 (230.8375, -88.75) -> (230.3375, -88.25) centre (230.3375, -88.75) ccw
  arc A314 (216.8375, -101.75) -> (217.3375, -102.25) centre (217.3375, -101.75) ccw
  arc A315 (230.3375, -102.25) -> (230.8375, -101.75) centre (230.3375, -101.75) ccw
  line L316 (253.0563, -88.25) -> (266.0562, -88.25)
  line L317 (253.0563, -102.25) -> (266.0562, -102.25)
  line L318 (252.5563, -88.75) -> (252.5563, -101.75)
  line L319 (266.5562, -88.75) -> (266.5562, -101.75)
  arc A316 (253.0563, -88.25) -> (252.5563, -88.75) centre (253.0563, -88.75) ccw
  arc A317 (266.5562, -88.75) -> (266.0562, -88.25) centre (266.0562, -88.75) ccw
  arc A318 (252.5563, -101.75) -> (253.0563, -102.25) centre (253.0563, -101.75) ccw
  arc A319 (266.0562, -102.25) -> (266.5562, -101.75) centre (266.0562, -101.75) ccw
  line L320 (244.6183, -89.25) -> (250.6182, -89.25)
  line L321 (244.6183, -104.25) -> (250.6182, -104.25)
  line L322 (244.1182, -89.75) -> (244.1182, -103.75)
  line L323 (251.1182, -89.75) -> (251.1182, -103.75)
  arc A320 (244.6183, -89.25) -> (244.1183, -89.75) centre (244.6183, -89.75) ccw
  arc A321 (251.1182, -89.75) -> (250.6182, -89.25) centre (250.6182, -89.75) ccw
  arc A322 (244.1183, -103.75) -> (244.6183, -104.25) centre (244.6183, -103.75) ccw
  arc A323 (250.6182, -104.25) -> (251.1182, -103.75) centre (250.6182, -103.75) ccw
  line L324 (268.4943, -89.25) -> (274.4943, -89.25)
  line L325 (268.4943, -104.25) -> (274.4943, -104.25)
  line L326 (267.9943, -89.75) -> (267.9943, -103.75)
  line L327 (274.9943, -89.75) -> (274.9943, -103.75)
  arc A324 (268.4943, -89.25) -> (267.9943, -89.75) centre (268.4943, -89.75) ccw
  arc A325 (274.9943, -89.75) -> (274.4943, -89.25) centre (274.4943, -89.75) ccw
  arc A326 (267.9943, -103.75) -> (268.4943, -104.25) centre (268.4943, -103.75) ccw
  arc A327 (274.4943, -104.25) -> (274.9943, -103.75) centre (274.4943, -103.75) ccw
  line L328 (312.5875, -88.25) -> (325.5875, -88.25)
  line L329 (312.5875, -102.25) -> (325.5875, -102.25)
  line L330 (312.0875, -88.75) -> (312.0875, -101.75)
  line L331 (326.0875, -88.75) -> (326.0875, -101.75)
  arc A328 (312.5875, -88.25) -> (312.0875, -88.75) centre (312.5875, -88.75) ccw
  arc A329 (326.0875, -88.75) -> (325.5875, -88.25) centre (325.5875, -88.75) ccw
  arc A330 (312.0875, -101.75) -> (312.5875, -102.25) centre (312.5875, -101.75) ccw
  arc A331 (325.5875, -102.25) -> (326.0875, -101.75) centre (325.5875, -101.75) ccw
  line L332 (5.4062, -107.3) -> (18.4063, -107.3)
  line L333 (5.4062, -121.3) -> (18.4063, -121.3)
  line L334 (4.9062, -107.8) -> (4.9062, -120.8)
  line L335 (18.9062, -107.8) -> (18.9062, -120.8)
  arc A332 (5.4062, -107.3) -> (4.9062, -107.8) centre (5.4062, -107.8) ccw
  arc A333 (18.9062, -107.8) -> (18.4062, -107.3) centre (18.4062, -107.8) ccw
  arc A334 (4.9062, -120.8) -> (5.4062, -121.3) centre (5.4062, -120.8) ccw
  arc A335 (18.4062, -121.3) -> (18.9063, -120.8) centre (18.4062, -120.8) ccw
  line L336 (29.2188, -107.3) -> (42.2188, -107.3)
  line L337 (29.2188, -121.3) -> (42.2188, -121.3)
  line L338 (28.7188, -107.8) -> (28.7188, -120.8)
  line L339 (42.7188, -107.8) -> (42.7188, -120.8)
  arc A336 (29.2188, -107.3) -> (28.7187, -107.8) centre (29.2188, -107.8) ccw
  arc A337 (42.7188, -107.8) -> (42.2188, -107.3) centre (42.2188, -107.8) ccw
  arc A338 (28.7188, -120.8) -> (29.2188, -121.3) centre (29.2188, -120.8) ccw
  arc A339 (42.2188, -121.3) -> (42.7188, -120.8) centre (42.2188, -120.8) ccw
  line L340 (53.0313, -107.3) -> (66.0312, -107.3)
  line L341 (53.0313, -121.3) -> (66.0312, -121.3)
  line L342 (52.5313, -107.8) -> (52.5313, -120.8)
  line L343 (66.5312, -107.8) -> (66.5312, -120.8)
  arc A340 (53.0313, -107.3) -> (52.5312, -107.8) centre (53.0313, -107.8) ccw
  arc A341 (66.5312, -107.8) -> (66.0312, -107.3) centre (66.0312, -107.8) ccw
  arc A342 (52.5313, -120.8) -> (53.0313, -121.3) centre (53.0313, -120.8) ccw
  arc A343 (66.0312, -121.3) -> (66.5312, -120.8) centre (66.0312, -120.8) ccw
  line L344 (124.4688, -107.3) -> (137.4688, -107.3)
  line L345 (124.4688, -121.3) -> (137.4688, -121.3)
  line L346 (123.9688, -107.8) -> (123.9688, -120.8)
  line L347 (137.9688, -107.8) -> (137.9688, -120.8)
  arc A344 (124.4688, -107.3) -> (123.9688, -107.8) centre (124.4688, -107.8) ccw
  arc A345 (137.9688, -107.8) -> (137.4688, -107.3) centre (137.4688, -107.8) ccw
  arc A346 (123.9688, -120.8) -> (124.4688, -121.3) centre (124.4688, -120.8) ccw
  arc A347 (137.4688, -121.3) -> (137.9688, -120.8) centre (137.4688, -120.8) ccw
  line L348 (77.9688, -108.3) -> (83.9688, -108.3)
  line L349 (77.9688, -123.3) -> (83.9688, -123.3)
  line L350 (77.4688, -108.8) -> (77.4688, -122.8)
  line L351 (84.4688, -108.8) -> (84.4688, -122.8)
  arc A348 (77.9688, -108.3) -> (77.4688, -108.8) centre (77.9688, -108.8) ccw
  arc A349 (84.4688, -108.8) -> (83.9688, -108.3) centre (83.9688, -108.8) ccw
  arc A350 (77.4688, -122.8) -> (77.9688, -123.3) centre (77.9688, -122.8) ccw
  arc A351 (83.9688, -123.3) -> (84.4687, -122.8) centre (83.9688, -122.8) ccw
  line L352 (177.9688, -108.3) -> (183.9688, -108.3)
  line L353 (177.9688, -123.3) -> (183.9688, -123.3)
  line L354 (177.4688, -108.8) -> (177.4688, -122.8)
  line L355 (184.4688, -108.8) -> (184.4688, -122.8)
  arc A352 (177.9688, -108.3) -> (177.4688, -108.8) centre (177.9688, -108.8) ccw
  arc A353 (184.4688, -108.8) -> (183.9688, -108.3) centre (183.9688, -108.8) ccw
  arc A354 (177.4688, -122.8) -> (177.9688, -123.3) centre (177.9688, -122.8) ccw
  arc A355 (183.9688, -123.3) -> (184.4688, -122.8) centre (183.9688, -122.8) ccw
  line L356 (195.9063, -107.3) -> (208.9062, -107.3)
  line L357 (195.9063, -121.3) -> (208.9062, -121.3)
  line L358 (195.4063, -107.8) -> (195.4063, -120.8)
  line L359 (209.4062, -107.8) -> (209.4062, -120.8)
  arc A356 (195.9063, -107.3) -> (195.4063, -107.8) centre (195.9063, -107.8) ccw
  arc A357 (209.4062, -107.8) -> (208.9062, -107.3) centre (208.9062, -107.8) ccw
  arc A358 (195.4063, -120.8) -> (195.9063, -121.3) centre (195.9063, -120.8) ccw
  arc A359 (208.9062, -121.3) -> (209.4062, -120.8) centre (208.9062, -120.8) ccw
  line L360 (219.7188, -107.3) -> (232.7188, -107.3)
  line L361 (219.7188, -121.3) -> (232.7188, -121.3)
  line L362 (219.2188, -107.8) -> (219.2188, -120.8)
  line L363 (233.2188, -107.8) -> (233.2188, -120.8)
  arc A360 (219.7188, -107.3) -> (219.2188, -107.8) centre (219.7188, -107.8) ccw
  arc A361 (233.2188, -107.8) -> (232.7188, -107.3) centre (232.7188, -107.8) ccw
  arc A362 (219.2188, -120.8) -> (219.7188, -121.3) centre (219.7188, -120.8) ccw
  arc A363 (232.7188, -121.3) -> (233.2188, -120.8) centre (232.7188, -120.8) ccw
  line L364 (243.5313, -107.3) -> (256.5313, -107.3)
  line L365 (243.5313, -121.3) -> (256.5313, -121.3)
  line L366 (243.0312, -107.8) -> (243.0312, -120.8)
  line L367 (257.0312, -107.8) -> (257.0312, -120.8)
  arc A364 (243.5313, -107.3) -> (243.0313, -107.8) centre (243.5313, -107.8) ccw
  arc A365 (257.0312, -107.8) -> (256.5312, -107.3) centre (256.5312, -107.8) ccw
  arc A366 (243.0313, -120.8) -> (243.5313, -121.3) centre (243.5313, -120.8) ccw
  arc A367 (256.5312, -121.3) -> (257.0312, -120.8) centre (256.5312, -120.8) ccw
  line L368 (267.3438, -107.3) -> (280.3438, -107.3)
  line L369 (267.3438, -121.3) -> (280.3438, -121.3)
  line L370 (266.8438, -107.8) -> (266.8438, -120.8)
  line L371 (280.8438, -107.8) -> (280.8438, -120.8)
  arc A368 (267.3438, -107.3) -> (266.8438, -107.8) centre (267.3438, -107.8) ccw
  arc A369 (280.8438, -107.8) -> (280.3438, -107.3) centre (280.3438, -107.8) ccw
  arc A370 (266.8438, -120.8) -> (267.3438, -121.3) centre (267.3438, -120.8) ccw
  arc A371 (280.3438, -121.3) -> (280.8438, -120.8) centre (280.3438, -120.8) ccw
  line L372 (293.5375, -107.3) -> (306.5375, -107.3)
  line L373 (293.5375, -121.3) -> (306.5375, -121.3)
  line L374 (293.0375, -107.8) -> (293.0375, -120.8)
  line L375 (307.0375, -107.8) -> (307.0375, -120.8)
  arc A372 (293.5375, -107.3) -> (293.0375, -107.8) centre (293.5375, -107.8) ccw
  arc A373 (307.0375, -107.8) -> (306.5375, -107.3) centre (306.5375, -107.8) ccw
  arc A374 (293.0375, -120.8) -> (293.5375, -121.3) centre (293.5375, -120.8) ccw
  arc A375 (306.5375, -121.3) -> (307.0375, -120.8) centre (306.5375, -120.8) ccw
  line L376 (312.5875, -107.3) -> (325.5875, -107.3)
  line L377 (312.5875, -121.3) -> (325.5875, -121.3)
  line L378 (312.0875, -107.8) -> (312.0875, -120.8)
  line L379 (326.0875, -107.8) -> (326.0875, -120.8)
  arc A376 (312.5875, -107.3) -> (312.0875, -107.8) centre (312.5875, -107.8) ccw
  arc A377 (326.0875, -107.8) -> (325.5875, -107.3) centre (325.5875, -107.8) ccw
  arc A378 (312.0875, -120.8) -> (312.5875, -121.3) centre (312.5875, -120.8) ccw
  arc A379 (325.5875, -121.3) -> (326.0875, -120.8) centre (325.5875, -120.8) ccw
  line L380 (331.6375, -107.3) -> (344.6375, -107.3)
  line L381 (331.6375, -121.3) -> (344.6375, -121.3)
  line L382 (331.1375, -107.8) -> (331.1375, -120.8)
  line L383 (345.1375, -107.8) -> (345.1375, -120.8)
  arc A380 (331.6375, -107.3) -> (331.1375, -107.8) centre (331.6375, -107.8) ccw
  arc A381 (345.1375, -107.8) -> (344.6375, -107.3) centre (344.6375, -107.8) ccw
  arc A382 (331.1375, -120.8) -> (331.6375, -121.3) centre (331.6375, -120.8) ccw
  arc A383 (344.6375, -121.3) -> (345.1375, -120.8) centre (344.6375, -120.8) ccw
  line L384 (410.182, 15.442) -> (-9.818, 15.442)
  arc A384 (-9.818, 15.442) -> (-20.318, 4.942) centre (-9.818, 4.942) ccw
  line L385 (-20.318, 4.942) -> (-20.318, -125.058)